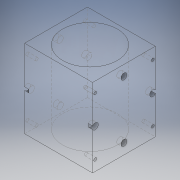
# Autodesk Inventor part: mid_block
Saved by Autodesk Inventor 2016 (Build 200138000, 138)
## iProperties
Created: 2016-02-26
Part Number: mid_block
Material: Generic
Document SubType Name: Modeling
Designer: USKHNGO
Density: 1 g/cm^3
Appearance: Default
Author: USKHNGO
Autodesk Inventor part; units mm, degrees
ref_plane "YZ Plane" through (0, 0, 0) normal (1, 0, 0) x (0, 1, 0)
ref_plane "XZ Plane" through (0, 0, 0) normal (0, 1, 0) x (-1, 0, 0)
ref_plane "XY Plane" through (0, 0, 0) normal (0, 0, 1) x (1, 0, 0)
sketch "Sketch1" plane through (0, 0, 0) normal (0, 1, 0) x (-1, 0, 0)
  line L0 (41.275, -38.1) -> (-41.275, -38.1)
  line L1 (-41.275, -38.1) -> (-41.275, 38.1)
  line L2 (-41.275, 38.1) -> (41.275, 38.1)
  line L3 (41.275, 38.1) -> (41.275, -38.1)
  circle A0 centre (0, 0) radius 4.5409
  dimension "d3" = 82.55
  dimension "d4" = 76.2
  constraints: 8 end point, 2 parallel, 1 centre point, 1 horizontal, 1 perpendicular
  measures "d3" distance of L1.end L2.end
  measures "d4" distance of L0.end L1.end
extrude "block" add sketch "Sketch1" along normal blind 95.25 contours L0 L1 L2 L3 | A0
sketch "Sketch2" plane through (0, 95.25, 0) normal (0, 1, 0) x (1, 0, 0)
  circle A0 centre (0, 0) radius 33.147
  dimension "d7" = 66.294
  constraints: 1 centre point, 1 coincident
  measures "d7" diameter of A0
extrude "hole" cut sketch "Sketch2" against normal blind 88.9
sketch "Sketch4" plane through (41.275, 0, 38.1) normal (1, 0, 0) x (0, 0, -1)
  line L0 (76.2, 85.6) -> (76.2, 9.4)
  line L1 (0, 9.4) -> (0, 85.6)
  line L2 (38.227, 85.727) -> (38.102, 85.727)
  line L3 (0, 0) -> (0, 95.25) projected
  line L4 (0, 47.625) -> (0, 47.375)
  line L5 (76.2, 0) -> (76.2, 95.25) projected
  line L6 (76.2, 47.625) -> (76.2, 47.5)
  line L7 (8.3242, 59.8735) -> (8.4492, 59.8735)
  line L8 (38.102, 85.727) -> (38.102, 82.552)
  circle A0 centre (38.102, 82.552) radius 3.683
  circle A1 centre (3.175, 47.625) radius 3.683
  circle A2 centre (38.102, 12.702) radius 3.683
  circle A3 centre (73.025, 47.5) radius 3.683
  line L9 (0, 47.625) -> (3.175, 47.625)
  line L10 (38.102, 82.425) -> (38.102, -13.1059)
  line L11 (3.175, 47.625) -> (115.5999, 47.625)
  circle A4 centre (73.025, 47.625) radius 0.0045
  point P0 (38.1, 0)
  dimension "d10" = 76.2
  dimension "d11" = 76.2
  dimension "d21" = 3.175
  dimension "d30" = 7.366
  dimension "d32" = 7.366
  dimension "d33" = 7.366
  dimension "d34" = 7.366
  dimension "d35" = 3.175
  constraints: 20 end point, 5 centre point, 3 point on line, 2 coincident, 2 horizontal, 2 midpoint, 2 vertical, 1 parallel, 1 perpendicular
  measures "d10" distance of L0.end L1.start
  measures "d11" distance of L0.start L0.end
  measures "d21" distance of L2.end L8.end
  measures "d30" diameter of A0
  measures "d32" diameter of A1
  measures "d33" diameter of A2
  measures "d34" diameter of A3
  measures "d35" distance of L4.start L9.end
extrude "Extrusion3" cut sketch "Sketch4" against normal blind 5.08
sketch "Sketch5" plane through (-41.275, 0, -38.1) normal (-1, 0, 0) x (0, 0, 1)
  line L0 (0, 85.6) -> (76.2, 85.6)
  line L1 (76.2, 85.6) -> (76.2, 9.4)
  line L2 (76.2, 9.4) -> (0, 9.4)
  line L3 (0, 9.4) -> (0, 85.6)
  line L4 (38.1, 85.6) -> (37.975, 85.6)
  line L5 (38.1, 9.4) -> (38.225, 9.4)
  line L6 (0, 0) -> (0, 95)
  line L7 (0, 47.5) -> (0, 47.375)
  line L8 (76.2, 0) -> (76.2, 95)
  line L9 (76.2, 47.5) -> (76.2, 47.375)
  line L10 (8.3242, 59.8735) -> (8.4492, 59.8735)
  line L11 (0, 47.375) -> (3.175, 47.375)
  line L12 (37.975, 85.6) -> (37.975, 82.425)
  line L13 (76.2, 47.375) -> (73.025, 47.375)
  line L14 (38.225, 9.4) -> (38.225, 12.575)
  circle A0 centre (3.175, 82.552) radius 1.7526
  circle A1 centre (73.025, 12.702) radius 1.7526
  circle A2 centre (3.175, 12.702) radius 1.7526
  circle A3 centre (73.025, 82.552) radius 1.7526
  point P0 (38.1, 0)
  point P1 (38.1, 0)
  dimension "d24" = 76.2
  dimension "d25" = 76.2
  dimension "d26" = 3.175
  dimension "d27" = 3.175
  dimension "d28" = 3.175
  dimension "d29" = 3.175
  dimension "d38" = 3.5052
  dimension "d39" = 3.5052
  dimension "d40" = 3.5052
  dimension "d41" = 3.5052
  constraints: 30 end point, 4 centre point, 4 midpoint, 4 point on line, 3 perpendicular, 2 horizontal, 2 parallel, 2 vertical
  measures "d24" distance of L1.end L2.end
  measures "d25" distance of L0.end L1.end
  measures "d26" distance of L11.start L11.end
  measures "d27" distance of L4.end L12.end
  measures "d28" distance of L9.end L13.end
  measures "d29" distance of L5.end L14.end
  measures "d38" diameter of A0
  measures "d39" diameter of A1
  measures "d40" diameter of A2
  measures "d41" diameter of A3
extrude "Extrusion4" cut sketch "Sketch5" against normal blind 11.43 contours A0 | A1 | A2 | A3
sketch "Sketch6" plane through (-41.275, 0, -38.1) normal (-1, 0, 0) x (0, 0, 1)
  circle A0 centre (38.098, 82.425) radius 3.683
  circle A1 centre (38.098, 82.425) radius 3.683
  circle A2 centre (3.175, 47.5) radius 3.683
  circle A3 centre (37.973, 12.575) radius 3.683
  circle A4 centre (37.973, 12.575) radius 3.683
  arc A5 (76.2, 49.3763) -> (76.2, 45.6433) centre (73.025, 47.5098) ccw
  circle A6 centre (73.025, 47.5098) radius 3.683
  line L0 (76.2, 95.0156) -> (0, 95.0156)
  line L1 (0, 0.0156) -> (0, 45.6334)
  line L2 (76.2, 0.0156) -> (76.2, 95.0156)
  line L3 (4.85, 95) -> (71.35, 95)
  line L4 (0, 0.0156) -> (76.2, 0.0156)
  arc A7 (0, 45.6334) -> (0, 49.3666) centre (3.175, 47.5) ccw projected
  point P0 (38.1, 0)
  point P1 (0, 95.0156)
  constraints: 7 centre point, 6 end point, 3 coincident, 2 point on circle, 6 other
extrude "Extrusion5" cut sketch "Sketch6" against normal blind 5.08
sketch "Sketch9" plane through (41.275, 0, 38.1) normal (1, 0, 0) x (0, 0, -1)
  circle A0 centre (3.175, 82.552) radius 1.7526 projected
  circle A1 centre (3.175, 82.552) radius 1.7526
  circle A2 centre (3.175, 12.702) radius 1.7526 projected
  circle A3 centre (3.175, 12.702) radius 1.7526
  circle A4 centre (73.025, 12.702) radius 1.7526 projected
  circle A5 centre (73.025, 12.702) radius 1.7526
  circle A6 centre (73.025, 82.552) radius 1.7526 projected
  circle A7 centre (73.025, 82.552) radius 1.7526
  point P0 (38.1, 0)
  constraints: 4 centre point, 4 coincident
extrude "Extrusion6" cut sketch "Sketch9" against normal blind 11.43
body "Solid1"
